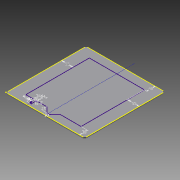
# Autodesk Inventor part: main_frame
Saved by Autodesk Inventor 2015 (Build 190159000, 159)
## iProperties
Created: 2014-12-25
Part Number: main_frame
Material: Generic
Document SubType Name: Modeling
Designer: X
Density: 1 g/cm^3
Appearance: Default
Author: X
Autodesk Inventor part; units mm, degrees
ref_plane "YZ Plane" through (0, 0, 0) normal (1, 0, 0) x (0, 1, 0)
ref_plane "XZ Plane" through (0, 0, 0) normal (0, 1, 0) x (-1, 0, 0)
ref_plane "XY Plane" through (0, 0, 0) normal (0, 0, 1) x (1, 0, 0)
sketch "Sketch1" plane through (0, 0, 0) normal (0, 0, 1) x (1, 0, 0)
  line L0 (7, 0) -> (363, 0)
  line L1 (370, 7) -> (370, 370)
  line L2 (363, 377) -> (7, 377)
  line L3 (0, 370) -> (0, 7)
  line L4 (7, 0) -> (0, 7)
  line L5 (-121.5053, 188.5) -> (511.4947, 188.5) construction
  line L6 (185, 402) -> (185, -38) construction
  line L7 (363, 0) -> (370, 7)
  line L8 (7, 377) -> (0, 370)
  line L9 (363, 377) -> (370, 370)
  point P0 (0, 0)
  point P1 (185, 377)
  point P2 (370, 188.5)
  dimension "height" = 370
  dimension "width" = 370
  dimension "Chamfer1" = 7
  dimension "Chamfer1ang" = 45
  constraints: 20 end point, 6 symmetric about line, 4 point on line, 2 horizontal, 2 midpoint, 2 parallel, 2 perpendicular
  measures "height" distance of L3.start point (0, 0)
  measures "width" distance between parallel lines of L3 L1
  measures "Chamfer1" distance of L0.start point (0, 0)
  measures "Chamfer1ang" angle of L0 L4
extrude "Extrusion1" add sketch "Sketch1" along normal blind 6
sketch "Sketch2" plane through (0, 0, 6) normal (0, 0, 1) x (1, 0, 0)
  line L0 (55, 337) -> (315, 337)
  line L1 (315, 337) -> (315, 38)
  line L2 (55, 38) -> (55, 337)
  line L3 (7, 377) -> (363, 377) projected
  line L4 (7, 0) -> (363, 0) projected
  line L5 (370, 370) -> (370, 7) projected
  line L6 (0, 370) -> (0, 7) projected
  line L7 (105, 34) -> (105, 18)
  line L8 (95, 18) -> (95, 34)
  line L9 (190, 13) -> (180, 13)
  line L10 (180, 13) -> (155, 38)
  line L11 (190, 13) -> (215, 38)
  line L12 (185, 422) -> (185, 5) construction
  arc A0 (95, 18) -> (105, 18) centre (100, 18) ccw
  line L13 (315, 38) -> (215, 38)
  line L14 (155, 38) -> (109, 38)
  line L15 (91, 38) -> (55, 38)
  line L16 (91, 38) -> (95, 34)
  line L17 (109, 38) -> (105, 34)
  point P0 (0, 0)
  point P1 (95, 38)
  point P2 (105, 38)
  point P3 (185, 337)
  point P4 (185, 13)
  point P5 (100, 13)
  dimension "top_dist" = 40
  dimension "Right_dist" = 55
  dimension "Left_dist" = 55
  dimension "width_triangle" = 10
  dimension "bot_dist" = 38
  dimension "width_slot" = 10
  dimension "position_slot" = 40
  dimension "Height_triangle" = 25
  dimension "d30" = 25
  dimension "d31" = 4
  dimension "d32" = 4
  dimension "d33" = 4
  dimension "d34" = 4
  constraints: 28 end point, 6 parallel, 6 point on line, 3 perpendicular, 3 point on circle, 2 collinear, 2 midpoint, 1 centre point, 1 horizontal, 1 tangent, 1 other
  measures "top_dist" distance between parallel lines of L3 L0
  measures "Right_dist" distance between parallel lines of L5 L1
  measures "Left_dist" distance between parallel lines of L6 L2
  measures "width_triangle" distance of L9.start L9.end
  measures "bot_dist" distance between parallel lines of L4 L13
  measures "width_slot" distance between parallel lines of L7 L8
  measures "position_slot" distance between parallel lines of L2 L8
  measures "Height_triangle" distance between parallel lines of L14 L9
  measures "d30" distance from line of L15 point (100, 13)
  measures "d31" distance of L15.start point (95, 38)
  measures "d32" distance of L8.end point (95, 38)
  measures "d33" distance of L14.end point (105, 38)
  measures "d34" distance of L7.start point (105, 38)
equation "\"d32\" = d31"
equation "\"d34\" = d33"
body "Solid1"
